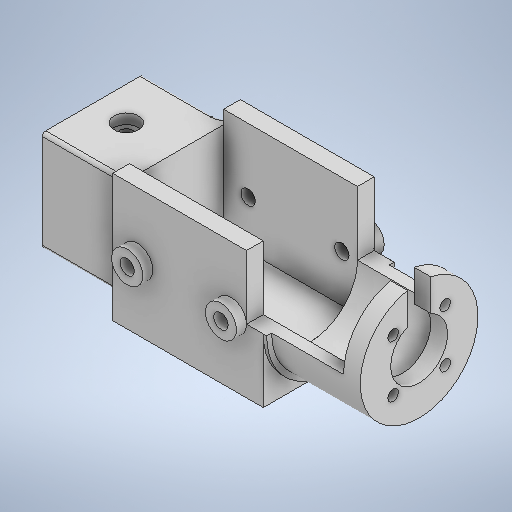
# Autodesk Inventor part: j4 motor mount
Saved by Autodesk Inventor 2025 (Build 290162000, 162)
## iProperties
Created: 2025-08-04
Part Number: j4 motor mount
Material: 一般
Document SubType Name: Modeling
Designer: gavin
Density: 1 g/cm^3
Appearance: 預設
Author: gavin
## iProperties of the stored document j4 motor mount_3D 列印.ipt
Created: 2025-08-05
Part Number: j4 motor mount_3D 列印
Material: 一般
Document SubType Name: Modeling
Designer: gavin
Density: 1 g/cm^3
Appearance: 預設
Author: gavin
Autodesk Inventor part; units mm, degrees
ref_plane "YZ Plane" through (0, 0, 0) normal (1, 0, 0) x (0, 1, 0)
ref_plane "XZ Plane" through (0, 0, 0) normal (0, 1, 0) x (-1, 0, 0)
ref_plane "XY Plane" through (0, 0, 0) normal (0, 0, 1) x (1, 0, 0)
sketch "草圖1" plane through (0, 0, 0) normal (1, 0, 0) x (0, 1, 0)
  line L0 (10.075, 10.075) -> (-10.075, 10.075)
  line L1 (-10.075, 10.075) -> (-10.075, -10.075)
  line L2 (-10.075, -10.075) -> (10.075, -10.075)
  line L3 (10.075, -10.075) -> (10.075, 10.075)
  line L4 (10.075, 10.075) -> (-10.075, -10.075) construction
  line L5 (-10.075, 10.075) -> (10.075, -10.075) construction
  line L6 (15.075, 15.075) -> (-15.075, 15.075)
  line L7 (-15.075, 15.075) -> (-15.075, -15.075)
  line L8 (-15.075, -15.075) -> (15.075, -15.075)
  line L9 (15.075, -15.075) -> (15.075, 15.075)
  point P0 (0, 0)
  dimension "d0" = 20.15
  dimension "d1" = 20.15
  dimension "d2" = 5
  constraints: 20 end point, 4 parallel, 2 midpoint, 2 perpendicular, 1 horizontal, 3 other
  measures "d0" distance of L2.end L1.end
  measures "d1" distance of L1.end L0.end
  measures "d2" distance between parallel lines of L3 L9
extrude "擠出1" add sketch "草圖1" along normal blind 20
sketch "草圖2" plane through (20, 0, 0) normal (1, 0, 0) x (0, 0, -1)
  line L0 (-15.075, -15.075) -> (15.075, -15.075) projected
  line L1 (15.075, -15.075) -> (15.075, 15.075) projected
  line L2 (15.075, 15.075) -> (-15.075, 15.075) projected
  line L3 (-15.075, 15.075) -> (-15.075, -15.075) projected
  line L4 (-10.075, 10.075) -> (10.075, 10.075) projected
  line L5 (10.075, 10.075) -> (10.075, -10.075) projected
  line L6 (10.075, -10.075) -> (-10.075, -10.075) projected
  line L7 (-10.075, -10.075) -> (-10.075, 10.075) projected
  point P0 (0, 0)
extrude "擠出2" add sketch "草圖2" along normal blind 5 contours L3 L2 L1 L0 | L4 L5 L6 L7
sketch "草圖3" plane through (25, 0, 0) normal (1, 0, 0) x (0, 0, -1)
  line L0 (-14.075, -14.075) -> (14.075, -14.075)
  line L1 (14.075, -14.075) -> (14.075, 14.075)
  line L2 (14.075, 14.075) -> (-14.075, 14.075)
  line L3 (-14.075, 14.075) -> (-14.075, -14.075)
  line L4 (-14.075, -14.075) -> (14.075, 14.075) construction
  line L5 (14.075, -14.075) -> (-14.075, 14.075) construction
  line L6 (-19.075, 19.075) -> (19.075, 19.075)
  line L7 (19.075, 19.075) -> (19.075, -19.075)
  line L8 (19.075, -19.075) -> (-19.075, -19.075)
  line L9 (-19.075, -19.075) -> (-19.075, 19.075)
  line L10 (-14.075, 14.075) -> (-14.075, 19.075)
  line L11 (14.075, 14.075) -> (14.075, 19.075)
  point P0 (0, 0)
  dimension "d7" = 28.15
  dimension "d8" = 28.15
  dimension "d9" = 5
  constraints: 24 end point, 4 parallel, 4 perpendicular, 2 midpoint, 2 point on line, 1 horizontal, 3 other
  measures "d7" distance of L2.end L1.end
  measures "d8" distance of L1.end L0.end
  measures "d9" distance between parallel lines of L2 L6
extrude "擠出3" add sketch "草圖3" along normal blind 40 contours L0 L1 L11 L6 L7 L8 L9 L10 L3
sketch "草圖4" plane through (65, 0, 0) normal (1, 0, 0) x (0, 0, -1)
  line L0 (14.075, -14.075) -> (-14.075, -14.075) projected
  line L1 (-14.075, -14.075) -> (-14.075, 19.075) projected
  line L2 (-14.075, 19.075) -> (-19.075, 19.075) projected
  line L3 (-19.075, 19.075) -> (-19.075, -19.075) projected
  line L4 (-19.075, -19.075) -> (19.075, -19.075) projected
  line L5 (19.075, -19.075) -> (19.075, 19.075) projected
  line L6 (19.075, 19.075) -> (14.075, 19.075) projected
  line L7 (14.075, 19.075) -> (14.075, -14.075) projected
  line L8 (-19.075, 0) -> (19.075, 0)
  point P0 (0, 0)
  constraints: 2 end point, 2 midpoint, 1 horizontal
extrude "擠出4" add sketch "草圖4" along normal blind 5 contours L7 L8 L5 L4 L3 L1 L0 | L0 L1 L8 L7
sketch "草圖5" plane through (70, 0, 0) normal (1, 0, 0) x (0, 0, -1)
  circle A0 centre (0, 0) radius 14.075
  dimension "d14" = 28.15
  constraints: 1 centre point, 1 coincident
  measures "d14" diameter of A0
extrude "擠出5" cut sketch "草圖5" against normal up to surface (5 mm away)
sketch "草圖6" plane through (70, 0, 0) normal (1, 0, 0) x (0, 0, -1)
  arc A0 (-14.075, 0) -> (14.075, 0) centre (0, 0) ccw projected
  arc A1 (-17.575, 0) -> (17.575, 0) centre (0, 0) ccw
  line L0 (-17.575, 0) -> (-14.075, 0)
  line L1 (14.075, 0) -> (17.575, 0)
  dimension "d37" = 17.575
  constraints: 4 end point, 2 point on circle, 1 centre point, 1 collinear, 1 horizontal
  measures "d37" radius of A1
extrude "擠出6" add sketch "草圖6" along normal blind 22.5
sketch "草圖7" plane through (92.5, 0, 0) normal (1, 0, 0) x (0, 0, -1)
  circle A0 centre (0, 0) radius 17.575
  circle A1 centre (0, 0) radius 8.5
  dimension "d20" = 17
  dimension "d36" = 35.15
  constraints: 2 centre point, 2 coincident
  measures "d20" diameter of A1
  measures "d36" diameter of A0
extrude "擠出7" add sketch "草圖7" along normal blind 5
sketch "草圖8" plane through (97.5, 0, 0) normal (1, 0, 0) x (0, 0, -1)
  circle A0 centre (0, 0) radius 11 construction
  line L0 (0, 0) -> (7.7782, 7.7782) construction
  line L1 (0, 0) -> (11, 0) construction
  circle A1 centre (7.7782, 7.7782) radius 1.6
  circle A2 centre (-7.7782, 7.7782) radius 1.6
  circle A3 centre (-7.7782, -7.7782) radius 1.6
  circle A4 centre (7.7782, -7.7782) radius 1.6
  dimension "d23" = 22
  dimension "d24" = 45
  dimension "d25" = 3.2
  dimension "d28" = 360
  constraints: 4 centre point, 4 end point, 2 coincident, 1 equal length, 1 horizontal, 12 other
  measures "d24" angle of L1 L0
  measures "d25" diameter of A1
extrude "擠出8" cut sketch "草圖8" against normal up to surface (5 mm away)
sketch "草圖9" plane through (97.5, 0, 0) normal (1, 0, 0) x (0, 0, -1)
  circle A0 centre (-7.7782, 7.7782) radius 1.6 projected
  circle A1 centre (-7.7782, -7.7782) radius 1.6 projected
  circle A2 centre (7.7782, 7.7782) radius 1.6 projected
  circle A3 centre (7.7782, -7.7782) radius 1.6 projected
  circle A4 centre (0, 0) radius 17.575 projected
  circle A5 centre (0, 0) radius 8.5 projected
  line L0 (-3.5, 17.223) -> (-3.5, 7.746)
  line L1 (3.5, 17.223) -> (3.5, 7.746)
  dimension "d32" = 7
  dimension "d33" = 3.5
  constraints: 4 end point, 4 point on circle, 2 vertical
  measures "d32" distance between parallel lines of L1 L0
  measures "d33" distance from line of A5.centre L1
extrude "擠出9" cut sketch "草圖9" against normal up to surface (5 mm away) contours L1 A5 L0 A4 picked at (2.1546, 14.356)
sketch "草圖12" plane through (70, 0, 0) normal (1, 0, 0) x (0, 0, -1)
  arc A0 (-17.575, 0) -> (17.575, 0) centre (0, 0) ccw projected
  line L0 (-17.575, 0) -> (-19.075, 0) projected
  line L1 (-19.075, 0) -> (-19.075, -19.075) projected
  line L2 (-19.075, -19.075) -> (19.075, -19.075) projected
  line L3 (19.075, -19.075) -> (19.075, 0) projected
  line L4 (19.075, 0) -> (17.575, 0) projected
extrude "擠出11" cut sketch "草圖12" against normal up to surface (5 mm away)
sketch "草圖13" plane through (65, 0, 0) normal (1, 0, 0) x (0, 0, -1)
  arc A0 (-3.5, 17.223) -> (3.5, 17.223) centre (0, 0) ccw projected
  line L0 (14.075, 0) -> (17.575, 0) projected
  arc A1 (14.075, -10.525) -> (17.575, 0) centre (0, 0) ccw projected
  line L1 (14.075, -10.525) -> (14.075, -14.075) projected
  line L2 (14.075, -14.075) -> (10.525, -14.075) projected
  arc A2 (-10.525, -14.075) -> (10.525, -14.075) centre (0, 0) ccw projected
  line L3 (-10.525, -14.075) -> (-14.075, -14.075) projected
  line L4 (-14.075, -14.075) -> (-14.075, -10.525) projected
  arc A3 (-17.575, 0) -> (-14.075, -10.525) centre (0, 0) ccw projected
  line L5 (-17.575, 0) -> (-14.075, 0) projected
  line L6 (-14.075, 0) -> (-14.075, 19.075) projected
  line L7 (-14.075, 19.075) -> (-19.075, 19.075) projected
  line L8 (-19.075, 19.075) -> (-19.075, -19.075) projected
  line L9 (19.075, -19.075) -> (-19.075, -19.075) projected
  line L10 (19.075, -19.075) -> (19.075, 19.075) projected
  line L11 (19.075, 19.075) -> (14.075, 19.075) projected
  line L12 (14.075, 19.075) -> (14.075, 0) projected
  line L13 (19.075, 0) -> (-19.075, 0)
  arc A4 (-3.7987, 18.6929) -> (3.7987, 18.6929) centre (0, 0) ccw
  point P0 (-17.575, 0)
  constraints: 2 end point, 2 midpoint, 2 point on circle, 1 centre point, 1 tangent
extrude "擠出12" add sketch "草圖13" along normal blind 5 contours A0 L4 A4 L13 | A0 L3 A4 L4 | A4 L4 L3 L9 L8 | A0 L2 A4 L3 | A4 L3 L4 | A0 L1 A4 L2 | L13 A4 L1 A0 | A4 L2 L1 L10 L9 | A4 L1 L2
fillet "圓角1" radius 4 3 edges at (25, 0, 15.075) (25, -15.075, 0) (25, 0, -15.075)
sketch "草圖14" plane through (70, 0, 0) normal (1, 0, 0) x (0, 0, -1)
  arc A0 (-3.5, 17.223) -> (3.5, 17.223) centre (0, 0) ccw projected
  line L0 (-19.075, -19.075) -> (19.075, -19.075) projected
  line L1 (19.075, -19.075) -> (19.075, 0) projected
  line L2 (19.075, 0) -> (17.575, 0) projected
  arc A1 (-17.575, 0) -> (17.575, 0) centre (0, 0) ccw projected
  line L3 (-17.575, 0) -> (-19.075, 0) projected
  line L4 (-19.075, 0) -> (-19.075, -19.075) projected
  arc A2 (-3.7987, 18.6929) -> (3.7987, 18.6929) centre (0, 0) ccw
  constraints: 2 point on circle, 1 centre point
extrude "擠出13" add sketch "草圖14" along normal blind 1 contours A0 L2 A2 L3
fillet "圓角2" radius 1 8 edges at (23.8285, 15.075, 16.2465) (10.5, 15.075, 15.075) (23.8285, -16.2465, 16.2465) (10.5, -15.075, 15.075) (23.8285, 15.075, -16.2465) (10.5, 15.075, -15.075) (23.8285, -16.2465, -16.2465) (10.5, -15.075, -15.075)
sketch "草圖15" plane through (25, 15.075, 14.075) normal (0, 1, 0) x (1, 0, 0)
  line L0 (-25, 4) -> (-25, 24.15) projected
  line L1 (-25, 24.15) -> (-5, 24.15) projected
  line L2 (-5, 4) -> (-5, 24.15) projected
  line L3 (-25, 4) -> (-5, 4) projected
  circle A0 centre (-15, 14.075) radius 2.1
  point P0 (-25, 14.075)
  dimension "d48" = 4.2
  constraints: 1 centre point
  measures "d48" diameter of A0
extrude "擠出14" cut sketch "草圖15" against normal through all contours A0
sketch "草圖16" plane through (25, 15.075, 14.075) normal (0, 1, 0) x (1, 0, 0)
  circle A0 centre (-15, 14.075) radius 2.1 projected
  circle A1 centre (-15, 14.075) radius 3.65
  point P0 (-25, 14.075)
  dimension "d51" = 7.3
  constraints: 1 centre point, 1 coincident
  measures "d51" diameter of A1
extrude "擠出15" cut sketch "草圖16" against normal blind 3 contours A0 | A1
mirror "鏡射1" about plane through (0, 0, 0) normal (0, 1, 0) of "擠出15"
sketch "草圖17" plane through (25, 19.075, 19.075) normal (0, 0, 1) x (1, 0, 0)
  line L0 (40, 0) -> (40, -19.075) projected
  line L1 (0, 0) -> (40, 0) projected
  line L2 (0, 0) -> (0, -5) projected
  line L3 (0, -5) -> (0, -38.15) projected
  line L4 (0, -38.15) -> (45, -38.15) projected
  line L5 (45, -19.075) -> (45, -38.15) projected
  line L6 (40, -19.075) -> (45, -19.075) projected
  circle A0 centre (7.335, -19.075) radius 2.165
  circle A1 centre (35.335, -19.075) radius 2.165
  circle A2 centre (35.335, -19.075) radius 4.665
  circle A3 centre (7.335, -19.075) radius 4.665
  line L7 (40, 0) -> (40, -19.075) projected
  point P0 (-25, -19.075)
  dimension "d54" = 4.33
  dimension "d55" = 4.33
  dimension "d56" = 28
  dimension "d57" = 2.5
  dimension "d58" = 2.5
  constraints: 4 centre point, 1 horizontal alignment, 1 tangent
  measures "d54" diameter of A0
  measures "d55" diameter of A1
  measures "d56" distance of A1.centre A0.centre
  measures "d57" radial gap between concentric circles of A1 A2
  measures "d58" radial gap between concentric circles of A0 A3
extrude "擠出16" add sketch "草圖17" along normal blind 3 contours A2 | A3
sketch "草圖18" plane through (32.335, 0, 19.075) normal (0, 0, 1) x (1, 0, 0)
  circle A0 centre (0, 0) radius 2.165 projected
  circle A1 centre (28, 0) radius 2.165 projected
  point P0 (-32.335, 0)
extrude "擠出17" cut sketch "草圖18" against normal up to surface (5 mm away)
mirror "鏡射2" about plane through (0, 0, 0) normal (0, 0, 1) of "擠出16", "擠出17"
